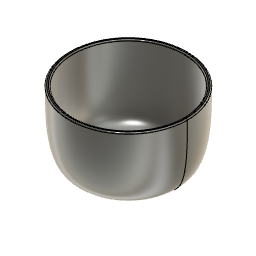
Bowl (Autodesk Fusion 360 design; units mm, degrees)
Autodesk Fusion 360 part; units mm, degrees
sketch "Sketch1" plane through (0, 0, 0) normal (0, 1, 0) x (1, 0, 0) in component "Component"
  line L0 (0, 0) -> (25, 0) construction
  line L1 (25, 0) -> (25, -50) construction
  line L2 (25, -50) -> (0, -50) construction
  line L3 (0, -50) -> (0, 0) construction
  spline S0 degree 5 poles (0, 0) (0.808, 0.0114) (2.3904, 0.0232) (4.663, 0.0085) (7.4897, -0.0768) (10.6759, -0.3012) (13.5055, -0.6649) (15.973, -1.2068) (18.0812, -1.9881) (19.8486, -3.0988) (21.3033, -4.6395) (22.4773, -6.7037) (23.4016, -9.3548) (24.103, -12.6168) (24.6036, -16.4912) (24.92, -20.966) (25.035, -25.0129) (25.0464, -28.3044) (25.021, -30.6119) (25, -31.7939) knots 0 0 0 0 0 0 0.066667 0.133333 0.2 0.266667 0.333333 0.4 0.466667 0.533333 0.6 0.666667 0.733333 0.8 0.866667 0.933333 1 1 1 1 1 1
  spline S1 degree 3 poles (0.0211, -1.4999) (5.0231, -1.4296) (9.2433, -1.5904) (12.518, -2.0842) (14.7348, -2.4185) (16.4853, -2.9122) (17.7973, -3.6623) (19.0702, -4.3899) (19.9982, -5.3482) (20.8052, -6.9542) (21.8468, -9.0268) (22.5978, -12.2188) (23.036, -16.502) (23.4594, -20.6395) (23.6069, -25.759) (23.5002, -31.7673) knots 0 0 0 0 0.25 0.25 0.25 0.419239 0.419239 0.419239 0.58342 0.58342 0.58342 0.795312 0.795312 0.795312 1 1 1 1
  line L4 (0, 0) -> (0.0211, -1.4999)
  line L5 (25, -31.7939) -> (23.5002, -31.7673)
  point P0 (16.0185, -1.307)
  point P1 (22, -6)
  dimension "d1" = 25
  dimension "d2" = 50
  dimension "d3" = 1.5
  constraint horizontal L0
  constraint vertical L1
  constraint horizontal L2
  constraint vertical L3
  constraint coincident L0.start L3.end
  constraint coincident L3 S1.start
  constraint coincident L1 S0.end
  measures "d1" distance of L0.start L0.end
  measures "d2" distance of L0.start L2.end
revolve "Revolve1" add sketch "Sketch1" angle 360 about axis through (0, 0, 50) along (0, 0, -1) in component "Component"
fillet "Fillet1" radius 0.5 2 edges at (-21.9099, -8.498, 31.7673) (-23.3082, -9.0404, 31.7939) in component "Component"
component "Component" placed x (1, 0, 0) y (0, 1, 0) z (0, 0, 1) at (0, 0, 0)
